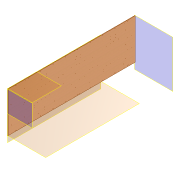
# Autodesk Inventor part: Top_Backboard
Saved by Autodesk Inventor 2018.1 (Build 221171000, 171)
## iProperties
Created: 2019-03-15
Part Number: Top_Backboard
Material: Wood (Cherry)
Document SubType Name: Modeling
Designer: James
Density: 0.63 g/cm^3
Appearance: Cherry - Natural Low Gloss
Mass: 60746.4 g
Surface Area: 108363 cm^2
Volume: 79929.5 cm^3
Author: James
Autodesk Inventor part; units mm, degrees
ref_plane "YZ Plane" through (0, 0, 0) normal (1, 0, 0) x (0, 1, 0)
ref_plane "XZ Plane" through (0, 0, 0) normal (0, 1, 0) x (-1, 0, 0)
ref_plane "XY Plane" through (0, 0, 0) normal (0, 0, 1) x (1, 0, 0)
derived "Top_Skeleton.ipt"
ref_plane "Work Plane1" through (0, 0, 0) normal (0, 0, 1) x (1, 0, 0)
ref_plane "Work Plane2" through (0, 0, 0) normal (0, 1, 0) x (-1, 0, 0)
ref_plane "Work Plane3" through (0, 0, 0) normal (1, 0, 0) x (0, 1, 0)
ref_plane "Work Plane4" through (0, 4100, 0) normal (0, 1, 0) x (-1, 0, 0)
ref_plane "Work Plane5" through (0, 0, -1300) normal (0, 0, 1) x (1, 0, 0)
sketch "Sketch2" plane through (0, 0, 0) normal (1, 0, 0) x (0, 1, 0)
  line L0 (0, 300) -> (0, -1800) projected
  line L1 (-820, 0) -> (4920, 0) projected
  line L2 (-820, -1300) -> (4920, -1300) projected
  line L3 (4100, 300) -> (4100, -1800) projected
  line L4 (0, 0) -> (4100, 0)
  line L5 (4100, 0) -> (4100, -1300)
  line L6 (4100, -1300) -> (0, -1300)
  line L7 (0, -1300) -> (0, 0)
  constraints: 8 end point, 4 point on line, 2 parallel, 1 horizontal, 1 perpendicular
extrude "Extrusion2" add sketch "Sketch2" along normal blind 15
sketch "Sketch3" plane through (15, 0, 0) normal (1, 0, 0) x (0, 0, -1)
  line L0 (1300, 4100) -> (0, 4100) projected
  line L1 (0, 4100) -> (0, 0) projected
  point P0 (487.5, 3991.5)
  point P1 (487.5, 3841.5)
  point P2 (822.5, 3841.5)
  point P3 (822.5, 3991.5)
  point P4 (487.5, 2881.3)
  point P5 (772.5, 2881.3)
  point P6 (772.5, 2731.3)
  point P7 (487.5, 2731.3)
  point P8 (487.5, 1771.1)
  point P9 (722.5, 1771.1)
  point P10 (722.5, 1621.1)
  point P11 (487.5, 1621.1)
  point P12 (487.5, 660.9)
  point P13 (672.5, 660.9)
  point P14 (672.5, 510.9)
  point P15 (487.5, 510.9)
  dimension "d7" = 150
  dimension "d8" = 335
  dimension "d16" = 150
  dimension "d17" = 150
  dimension "d18" = 150
  dimension "d19" = 285
  dimension "d20" = 235
  dimension "d21" = 185
  dimension "d22" = 108.5
  dimension "d23" = 487.5
  dimension "d24" = 1110.2
  dimension "d25" = 1110.2
  dimension "d26" = 1110.2
  constraints: 11 vertical alignment, 8 horizontal alignment
  measures "d7" distance of point (487.5, 3841.5) point (487.5, 3991.5)
  measures "d8" distance of point (822.5, 3991.5) point (487.5, 3991.5)
  measures "d16" distance of point (487.5, 2731.3) point (487.5, 2881.3)
  measures "d17" distance of point (487.5, 1621.1) point (487.5, 1771.1)
  measures "d18" distance of point (487.5, 510.9) point (487.5, 660.9)
  measures "d19" distance of point (772.5, 2881.3) point (487.5, 2881.3)
  measures "d20" distance of point (722.5, 1771.1) point (487.5, 1771.1)
  measures "d21" distance of point (672.5, 660.9) point (487.5, 660.9)
  measures "d22" distance from line of L0 point (487.5, 3991.5)
  measures "d23" distance from line of L1 point (487.5, 3991.5)
  measures "d24" vertical distance of point (772.5, 2881.3) point (822.5, 3991.5)
  measures "d25" vertical distance of point (722.5, 1771.1) point (772.5, 2881.3)
  measures "d26" vertical distance of point (672.5, 660.9) point (722.5, 1771.1)
hole "Selection Holes" at (15, 3991.5, -487.5) at (15, 3841.5, -487.5) at (15, 3841.5, -822.5) at (15, 3991.5, -822.5) at (15, 2881.3, -772.5) at (15, 2731.3, -772.5) at (15, 2731.3, -487.5) at (15, 2881.3, -487.5) at (15, 1771.1, -487.5) at (15, 1621.1, -487.5) at (15, 1621.1, -722.5) at (15, 1771.1, -722.5) at (15, 660.9, -487.5) at (15, 660.9, -672.5) at (15, 510.9, -672.5) at (15, 510.9, -487.5) direction (-1, 0, 0) diameter 4.5 end through all clearance for "Flat Head Machine Screw" size "M4" standard "Ansi Metric M Profile"
sketch "Sketch4" plane through (15, 0, 0) normal (1, 0, 0) x (0, 0, -1)
  circle A0 centre (672.5, 510.9) radius 2.25 projected
  circle A1 centre (487.5, 660.9) radius 2.25 projected
  circle A2 centre (722.5, 1621.1) radius 2.25 projected
  circle A3 centre (487.5, 1771.1) radius 2.25 projected
  circle A4 centre (487.5, 2731.3) radius 2.25 projected
  circle A5 centre (772.5, 2881.3) radius 2.25 projected
  circle A6 centre (822.5, 3841.5) radius 2.25 projected
  circle A7 centre (487.5, 3991.5) radius 2.25 projected
  circle A8 centre (487.5, 3841.5) radius 2.25 projected
  circle A9 centre (822.5, 3991.5) radius 2.25 projected
  circle A10 centre (772.5, 2731.3) radius 2.25 projected
  circle A11 centre (487.5, 2881.3) radius 2.25 projected
  circle A12 centre (487.5, 1621.1) radius 2.25 projected
  circle A13 centre (722.5, 1771.1) radius 2.25 projected
  circle A14 centre (672.5, 660.9) radius 2.25 projected
  circle A15 centre (487.5, 510.9) radius 2.25 projected
  line L0 (0, 0) -> (1300, 0) projected
  line L1 (1300, 0) -> (1300, 4100) projected
  line L2 (1300, 4100) -> (0, 4100) projected
  line L3 (0, 4100) -> (0, 0) projected
  point P0 (380, 3563)
  point P1 (935, 3563)
  point P2 (935, 3413)
  point P3 (380, 3413)
  point P4 (425, 2452.5)
  point P5 (885, 2452.5)
  point P6 (885, 2302.5)
  point P7 (425, 2302.5)
  point P8 (470, 1342.5)
  point P9 (835, 1342.5)
  point P10 (835, 1192.5)
  point P11 (470, 1192.5)
  dimension "d27" = 150
  dimension "d28" = 150
  dimension "d29" = 150
  dimension "d30" = 380
  dimension "d31" = 425
  dimension "d32" = 470
  dimension "d33" = 460
  dimension "d34" = 365
  dimension "d35" = 555
  dimension "d43" = 537
  dimension "d49" = 1110.5
  dimension "d50" = 1110
  constraints: 6 horizontal alignment, 6 vertical alignment
  measures "d27" distance of point (835, 1192.5) point (835, 1342.5)
  measures "d28" distance of point (885, 2452.5) point (885, 2302.5)
  measures "d29" distance of point (935, 3563) point (935, 3413)
  measures "d30" distance from line of L3 point (380, 3563)
  measures "d31" distance from line of point (425, 2452.5) L3
  measures "d32" distance from line of point (470, 1342.5) L3
  measures "d33" distance of point (885, 2452.5) point (425, 2452.5)
  measures "d34" distance of point (835, 1342.5) point (470, 1342.5)
  measures "d35" distance of point (935, 3563) point (380, 3563)
  measures "d43" distance from line of L2 point (935, 3563)
  measures "d49" vertical distance of point (885, 2452.5) point (935, 3563)
  measures "d50" vertical distance of point (835, 1342.5) point (885, 2452.5)
hole "Pancake Holes" at (15, 3563, -380) at (15, 3563, -935) at (15, 3413, -935) at (15, 3413, -380) at (15, 2452.5, -425) at (15, 2452.5, -885) at (15, 2302.5, -885) at (15, 2302.5, -425) at (15, 1342.5, -470) at (15, 1342.5, -835) at (15, 1192.5, -835) at (15, 1192.5, -470) direction (-1, 0, 0) diameter 4.5 end through all clearance for "Flat Head Machine Screw" size "M4" standard "Ansi Metric M Profile"
pattern_linear "Rectangular Pattern1" count 2 spacing 250 along (0, -1, 0) of "Pancake Holes"
sketch "Sketch5" plane through (15, 0, 0) normal (1, 0, 0) x (0, 0, -1)
  line L0 (1300, 0) -> (1300, 4100) projected
  line L1 (0, 4100) -> (0, 0) projected
  line L2 (-260, 4100) -> (1560, 4100) projected
  point P0 (25, 3850)
  point P1 (1275, 3850)
  dimension "d51" = 25
  dimension "d52" = 25
  dimension "d53" = 250
  constraints: 1 horizontal alignment
  measures "d51" distance from line of L0 point (1275, 3850)
  measures "d52" distance from line of L1 point (25, 3850)
  measures "d53" distance from line of point (25, 3850) L2
hole "Hole3" at (15, 3850, -25) at (15, 3850, -1275) direction (-1, 0, 0) diameter 4.496 end through all countersink diameter 8.433 countersink angle 82 clearance for "Flat Head Machine Screw (82)" size "#8" standard "Ansi Unified Screw Threads"
pattern_linear "Rectangular Pattern2" count 10 spacing 400 along (0, -1, 0) of "Hole3"
sketch "Sketch6" plane through (15, 0, 0) normal (1, 0, 0) x (0, 0, -1)
  line L0 (0, 4100) -> (0, 0) projected
  line L1 (-260, 4100) -> (1560, 4100) projected
  point P0 (250, 3800)
  point P1 (250, 2170)
  point P2 (250, 540)
  dimension "d64" = 250
  dimension "d65" = 300
  dimension "d76" = 1630
  dimension "d77" = 1630
  constraints: 2 vertical alignment
  measures "d64" distance from line of point (250, 3800) L0
  measures "d65" distance from line of point (250, 3800) L1
  measures "d76" distance of point (250, 2170) point (250, 3800)
  measures "d77" distance of point (250, 540) point (250, 2170)
hole "Hole4" at (15, 3800, -250) at (15, 2170, -250) at (15, 540, -250) direction (-1, 0, 0) diameter 4.496 end through all countersink diameter 8.433 countersink angle 82 clearance for "Flat Head Machine Screw (82)" size "#8" standard "Ansi Unified Screw Threads"
pattern_linear "Rectangular Pattern3" count 3 spacing 400 along (0, 0, -1) of "Hole4"
sketch "Sketch7" plane through (15, 0, 0) normal (1, 0, 0) x (0, 0, -1)
  circle A0 centre (1050, 2170) radius 4.2165 projected
  circle A1 centre (1050, 540) radius 4.2165 projected
  circle A2 centre (1050, 3800) radius 4.2165 projected
  circle A3 centre (650, 2170) radius 4.2165 projected
  circle A4 centre (650, 540) radius 4.2165 projected
  circle A5 centre (650, 3800) radius 4.2165 projected
  circle A6 centre (250, 2170) radius 4.2165 projected
  circle A7 centre (250, 3800) radius 4.2165 projected
  circle A8 centre (250, 540) radius 4.2165 projected
  circle A9 centre (25, 250) radius 4.2165 projected
  circle A10 centre (1275, 250) radius 4.2165 projected
  circle A11 centre (25, 650) radius 4.2165 projected
  circle A12 centre (1275, 650) radius 4.2165 projected
  circle A13 centre (25, 1050) radius 4.2165 projected
  circle A14 centre (1275, 1050) radius 4.2165 projected
  circle A15 centre (25, 1450) radius 4.2165 projected
  circle A16 centre (1275, 1450) radius 4.2165 projected
  circle A17 centre (25, 1850) radius 4.2165 projected
  circle A18 centre (1275, 1850) radius 4.2165 projected
  circle A19 centre (25, 2250) radius 4.2165 projected
  circle A20 centre (1275, 2250) radius 4.2165 projected
  circle A21 centre (25, 2650) radius 4.2165 projected
  circle A22 centre (1275, 2650) radius 4.2165 projected
  circle A23 centre (25, 3050) radius 4.2165 projected
  circle A24 centre (1275, 3050) radius 4.2165 projected
  circle A25 centre (25, 3450) radius 4.2165 projected
  circle A26 centre (1275, 3450) radius 4.2165 projected
  circle A27 centre (25, 3850) radius 4.2165 projected
  circle A28 centre (1275, 3850) radius 4.2165 projected
  circle A29 centre (835, 942.5) radius 2.25 projected
  circle A30 centre (470, 942.5) radius 2.25 projected
  circle A31 centre (835, 1092.5) radius 2.25 projected
  circle A32 centre (425, 2052.5) radius 2.25 projected
  circle A33 centre (885, 2202.5) radius 2.25 projected
  circle A34 centre (380, 3163) radius 2.25 projected
  circle A35 centre (935, 3313) radius 2.25 projected
  circle A36 centre (380, 3313) radius 2.25 projected
  circle A37 centre (935, 3163) radius 2.25 projected
  circle A38 centre (425, 2202.5) radius 2.25 projected
  circle A39 centre (885, 2052.5) radius 2.25 projected
  circle A40 centre (470, 1092.5) radius 2.25 projected
  circle A41 centre (835, 1192.5) radius 2.25 projected
  circle A42 centre (470, 1342.5) radius 2.25 projected
  circle A43 centre (885, 2302.5) radius 2.25 projected
  circle A44 centre (425, 2452.5) radius 2.25 projected
  circle A45 centre (935, 3413) radius 2.25 projected
  circle A46 centre (380, 3563) radius 2.25 projected
  circle A47 centre (935, 3563) radius 2.25 projected
  circle A48 centre (380, 3413) radius 2.25 projected
  circle A49 centre (885, 2452.5) radius 2.25 projected
  circle A50 centre (425, 2302.5) radius 2.25 projected
  circle A51 centre (835, 1342.5) radius 2.25 projected
  circle A52 centre (470, 1192.5) radius 2.25 projected
  circle A53 centre (672.5, 510.9) radius 2.25 projected
  circle A54 centre (487.5, 660.9) radius 2.25 projected
  circle A55 centre (722.5, 1621.1) radius 2.25 projected
  circle A56 centre (487.5, 1771.1) radius 2.25 projected
  circle A57 centre (487.5, 2731.3) radius 2.25 projected
  circle A58 centre (772.5, 2881.3) radius 2.25 projected
  circle A59 centre (822.5, 3841.5) radius 2.25 projected
  circle A60 centre (487.5, 3991.5) radius 2.25 projected
  circle A61 centre (487.5, 3841.5) radius 2.25 projected
  circle A62 centre (822.5, 3991.5) radius 2.25 projected
  circle A63 centre (772.5, 2731.3) radius 2.25 projected
  circle A64 centre (487.5, 2881.3) radius 2.25 projected
  circle A65 centre (487.5, 1621.1) radius 2.25 projected
  circle A66 centre (722.5, 1771.1) radius 2.25 projected
  circle A67 centre (672.5, 660.9) radius 2.25 projected
  circle A68 centre (487.5, 510.9) radius 2.25 projected
  line L0 (0, 0) -> (1300, 0) projected
  line L1 (1300, 0) -> (1300, 4100) projected
  line L2 (1300, 4100) -> (0, 4100) projected
  line L3 (0, 4100) -> (0, 0) projected
  point P0 (277.5, 3461.5)
  point P1 (277.5, 3311.5)
  point P2 (196.5, 3461.5)
  point P3 (196.5, 3311.5)
  point P4 (196.5, 2351.3)
  point P5 (277.5, 2351.3)
  point P6 (277.5, 2201.3)
  point P7 (196.5, 2201.3)
  point P8 (196.5, 1241.1)
  point P9 (277.5, 1241.1)
  point P10 (277.5, 1091.1)
  point P11 (196.5, 1091.1)
  dimension "d81" = 81
  dimension "d82" = 150
  dimension "d83" = 150
  dimension "d84" = 81
  dimension "d85" = 81
  dimension "d86" = 150
  dimension "d96" = 380
  dimension "d97" = 210
  dimension "d98" = 380
  dimension "d99" = 210
  dimension "d100" = 380
  dimension "d101" = 210
  constraints: 6 horizontal alignment, 6 vertical alignment
  measures "d81" distance of point (277.5, 3461.5) point (196.5, 3461.5)
  measures "d82" distance of point (196.5, 3311.5) point (196.5, 3461.5)
  measures "d83" distance of point (196.5, 2201.3) point (196.5, 2351.3)
  measures "d84" distance of point (277.5, 2351.3) point (196.5, 2351.3)
  measures "d85" distance of point (277.5, 1241.1) point (196.5, 1241.1)
  measures "d86" distance of point (196.5, 1241.1) point (196.5, 1091.1)
  measures "d96" vertical distance of point (277.5, 3461.5) A61.centre
  measures "d97" horizontal distance of A61.centre point (277.5, 3461.5)
  measures "d98" vertical distance of A57.centre point (277.5, 2351.3)
  measures "d99" horizontal distance of A57.centre point (277.5, 2351.3)
  measures "d100" vertical distance of A65.centre point (277.5, 1241.1)
  measures "d101" horizontal distance of A65.centre point (277.5, 1241.1)
hole "Hole5" at (15, 3461.5, -277.5) at (15, 3311.5, -277.5) at (15, 3461.5, -196.5) at (15, 3311.5, -196.5) at (15, 2351.3, -196.5) at (15, 2351.3, -277.5) at (15, 2201.3, -277.5) at (15, 2201.3, -196.5) at (15, 1241.1, -196.5) at (15, 1241.1, -277.5) at (15, 1091.1, -277.5) at (15, 1091.1, -196.5) direction (-1, 0, 0) diameter 4.5 end through all clearance for "Flat Head Machine Screw" size "M4" standard "Ansi Metric M Profile"
sketch "Sketch8" plane through (15, 0, 0) normal (1, 0, 0) x (0, 0, -1)
  circle A0 centre (277.5, 1091.1) radius 2.25 projected
  circle A1 centre (196.5, 1241.1) radius 2.25 projected
  circle A2 centre (277.5, 2201.3) radius 2.25 projected
  circle A3 centre (196.5, 2351.3) radius 2.25 projected
  circle A4 centre (196.5, 3461.5) radius 2.25 projected
  circle A5 centre (277.5, 3461.5) radius 2.25 projected
  circle A6 centre (277.5, 3311.5) radius 2.25 projected
  circle A7 centre (196.5, 3311.5) radius 2.25 projected
  circle A8 centre (277.5, 2351.3) radius 2.25 projected
  circle A9 centre (196.5, 2201.3) radius 2.25 projected
  circle A10 centre (277.5, 1241.1) radius 2.25 projected
  circle A11 centre (196.5, 1091.1) radius 2.25 projected
  circle A12 centre (1050, 2170) radius 4.2165 projected
  circle A13 centre (1050, 540) radius 4.2165 projected
  circle A14 centre (1050, 3800) radius 4.2165 projected
  circle A15 centre (650, 2170) radius 4.2165 projected
  circle A16 centre (650, 540) radius 4.2165 projected
  circle A17 centre (650, 3800) radius 4.2165 projected
  circle A18 centre (250, 2170) radius 4.2165 projected
  circle A19 centre (250, 3800) radius 4.2165 projected
  circle A20 centre (250, 540) radius 4.2165 projected
  circle A21 centre (25, 250) radius 4.2165 projected
  circle A22 centre (1275, 250) radius 4.2165 projected
  circle A23 centre (25, 650) radius 4.2165 projected
  circle A24 centre (1275, 650) radius 4.2165 projected
  circle A25 centre (25, 1050) radius 4.2165 projected
  circle A26 centre (1275, 1050) radius 4.2165 projected
  circle A27 centre (25, 1450) radius 4.2165 projected
  circle A28 centre (1275, 1450) radius 4.2165 projected
  circle A29 centre (25, 1850) radius 4.2165 projected
  circle A30 centre (1275, 1850) radius 4.2165 projected
  circle A31 centre (25, 2250) radius 4.2165 projected
  circle A32 centre (1275, 2250) radius 4.2165 projected
  circle A33 centre (25, 2650) radius 4.2165 projected
  circle A34 centre (1275, 2650) radius 4.2165 projected
  circle A35 centre (25, 3050) radius 4.2165 projected
  circle A36 centre (1275, 3050) radius 4.2165 projected
  circle A37 centre (25, 3450) radius 4.2165 projected
  circle A38 centre (1275, 3450) radius 4.2165 projected
  circle A39 centre (25, 3850) radius 4.2165 projected
  circle A40 centre (1275, 3850) radius 4.2165 projected
  circle A41 centre (835, 942.5) radius 2.25 projected
  circle A42 centre (470, 942.5) radius 2.25 projected
  circle A43 centre (835, 1092.5) radius 2.25 projected
  circle A44 centre (425, 2052.5) radius 2.25 projected
  circle A45 centre (885, 2202.5) radius 2.25 projected
  circle A46 centre (380, 3163) radius 2.25 projected
  circle A47 centre (935, 3313) radius 2.25 projected
  circle A48 centre (380, 3313) radius 2.25 projected
  circle A49 centre (935, 3163) radius 2.25 projected
  circle A50 centre (425, 2202.5) radius 2.25 projected
  circle A51 centre (885, 2052.5) radius 2.25 projected
  circle A52 centre (470, 1092.5) radius 2.25 projected
  circle A53 centre (835, 1192.5) radius 2.25 projected
  circle A54 centre (470, 1342.5) radius 2.25 projected
  circle A55 centre (885, 2302.5) radius 2.25 projected
  circle A56 centre (425, 2452.5) radius 2.25 projected
  circle A57 centre (935, 3413) radius 2.25 projected
  circle A58 centre (380, 3563) radius 2.25 projected
  circle A59 centre (935, 3563) radius 2.25 projected
  circle A60 centre (380, 3413) radius 2.25 projected
  circle A61 centre (885, 2452.5) radius 2.25 projected
  circle A62 centre (425, 2302.5) radius 2.25 projected
  circle A63 centre (835, 1342.5) radius 2.25 projected
  circle A64 centre (470, 1192.5) radius 2.25 projected
  circle A65 centre (672.5, 510.9) radius 2.25 projected
  circle A66 centre (487.5, 660.9) radius 2.25 projected
  circle A67 centre (722.5, 1621.1) radius 2.25 projected
  circle A68 centre (487.5, 1771.1) radius 2.25 projected
  circle A69 centre (487.5, 2731.3) radius 2.25 projected
  circle A70 centre (772.5, 2881.3) radius 2.25 projected
  circle A71 centre (822.5, 3841.5) radius 2.25 projected
  circle A72 centre (487.5, 3991.5) radius 2.25 projected
  circle A73 centre (487.5, 3841.5) radius 2.25 projected
  circle A74 centre (822.5, 3991.5) radius 2.25 projected
  circle A75 centre (772.5, 2731.3) radius 2.25 projected
  circle A76 centre (487.5, 2881.3) radius 2.25 projected
  circle A77 centre (487.5, 1621.1) radius 2.25 projected
  circle A78 centre (722.5, 1771.1) radius 2.25 projected
  circle A79 centre (672.5, 660.9) radius 2.25 projected
  circle A80 centre (487.5, 510.9) radius 2.25 projected
  line L0 (0, 0) -> (1300, 0) projected
  line L1 (1300, 0) -> (1300, 4100) projected
  line L2 (1300, 4100) -> (0, 4100) projected
  line L3 (0, 4100) -> (0, 0) projected
  point P0 (997, 3085.5)
  point P1 (1043, 3085.5)
  point P2 (947, 1974.5)
  point P3 (993, 1974.5)
  point P4 (897, 864.5)
  point P5 (943, 864.5)
  point P6 (747, 237)
  point P7 (793, 237)
  point P8 (872, 237)
  point P9 (918, 237)
  point P10 (997, 237)
  point P11 (1043, 237)
  point P12 (497, 237)
  point P13 (543, 237)
  point P14 (622, 237)
  point P15 (668, 237)
  dimension "d102" = 257
  dimension "d103" = 1014.5
  dimension "d104" = 46
  dimension "d105" = 46
  dimension "d106" = 46
  dimension "d107" = 46
  dimension "d108" = 46
  dimension "d109" = 46
  dimension "d110" = 2125.5
  dimension "d111" = 307
  dimension "d112" = 357
  dimension "d113" = 3235.5
  dimension "d121" = 3863
  dimension "d122" = 257
  dimension "d123" = 125
  dimension "d124" = 125
  dimension "d125" = 46
  dimension "d126" = 46
  dimension "d127" = 125
  dimension "d128" = 125
  constraints: 12 horizontal alignment
  measures "d102" distance from line of L1 point (1043, 3085.5)
  measures "d103" distance from line of L2 point (1043, 3085.5)
  measures "d104" distance of point (1043, 3085.5) point (997, 3085.5)
  measures "d105" distance of point (993, 1974.5) point (947, 1974.5)
  measures "d106" distance of point (943, 864.5) point (897, 864.5)
  measures "d107" distance of point (793, 237) point (747, 237)
  measures "d108" distance of point (918, 237) point (872, 237)
  measures "d109" distance of point (1043, 237) point (997, 237)
  measures "d110" distance from line of point (993, 1974.5) L2
  measures "d111" distance from line of point (993, 1974.5) L1
  measures "d112" distance from line of L1 point (943, 864.5)
  measures "d113" distance from line of L2 point (943, 864.5)
  measures "d121" distance from line of point (1043, 237) L2
  measures "d122" distance from line of point (1043, 237) L1
  measures "d123" distance of point (1043, 237) point (918, 237)
  measures "d124" distance of point (918, 237) point (793, 237)
  measures "d125" distance of point (668, 237) point (622, 237)
  measures "d126" distance of point (543, 237) point (497, 237)
  measures "d127" distance of point (747, 237) point (622, 237)
  measures "d128" distance of point (622, 237) point (497, 237)
hole "Hole6" at (15, 3085.5, -997) at (15, 3085.5, -1043) at (15, 1974.5, -947) at (15, 1974.5, -993) at (15, 864.5, -897) at (15, 864.5, -943) direction (-1, 0, 0) diameter 3.4 end through all clearance for "Flat Head Machine Screw" size "M3" standard "Ansi Metric M Profile"
sketch "Sketch9" plane through (15, 0, 0) normal (1, 0, 0) x (0, 0, -1)
  circle A0 centre (722.5, 1771.1) radius 2.25 projected
  point P0 (0, 0)
  point P1 (1172.5, 971.1)
  dimension "d129" = 450
  dimension "d130" = 800
  measures "d129" horizontal distance of A0.centre point (1172.5, 971.1)
  measures "d130" vertical distance of point (1172.5, 971.1) A0.centre
hole "Hole7" at (15, 971.1, -1172.5) direction (-1, 0, 0) diameter 9 end through all clearance for "Flat Head Machine Screw" size "M8" standard "Ansi Metric M Profile"
sketch "Sketch10" plane through (15, 0, 0) normal (1, 0, 0) x (0, 0, -1)
  circle A0 centre (1172.5, 971.1) radius 4.5 projected
  circle A1 centre (822.5, 3841.5) radius 2.25 projected
  circle A2 centre (772.5, 2731.3) radius 2.25 projected
  circle A3 centre (722.5, 1621.1) radius 2.25 projected
  point P0 (0, 0)
  point P1 (1072.5, 1171.1)
  point P2 (1112.5, 1171.1)
  point P3 (1152.5, 1171.1)
  point P4 (730, 1531.1)
  point P5 (780, 2641.3)
  point P6 (830, 3751.5)
  point P7 (1059.5, 1501.1)
  point P8 (1085.5, 1501.1)
  point P9 (1096.5, 2611.3)
  point P10 (1122.5, 2611.3)
  point P11 (1136.5, 3721.5)
  point P12 (1162.5, 3721.5)
  dimension "d138" = 100
  dimension "d139" = 40
  dimension "d140" = 40
  dimension "d141" = 200
  dimension "d149" = 90
  dimension "d150" = 7.5
  dimension "d151" = 90
  dimension "d152" = 7.5
  dimension "d153" = 90
  dimension "d154" = 7.5
  dimension "d155" = 26
  dimension "d156" = 26
  dimension "d157" = 26
  dimension "d158" = 13
  dimension "d159" = 16
  dimension "d160" = 10
  dimension "d161" = 30
  dimension "d162" = 30
  dimension "d163" = 30
  constraints: 5 horizontal alignment
  measures "d138" horizontal distance of A0.centre point (1072.5, 1171.1)
  measures "d139" distance of point (1072.5, 1171.1) point (1112.5, 1171.1)
  measures "d140" distance of point (1152.5, 1171.1) point (1112.5, 1171.1)
  measures "d141" vertical distance of A0.centre point (1152.5, 1171.1)
  measures "d149" vertical distance of point (730, 1531.1) A3.centre
  measures "d150" horizontal distance of A3.centre point (730, 1531.1)
  measures "d151" vertical distance of point (780, 2641.3) A2.centre
  measures "d152" horizontal distance of point (780, 2641.3) A2.centre
  measures "d153" vertical distance of A1.centre point (830, 3751.5)
  measures "d154" horizontal distance of point (830, 3751.5) A1.centre
  measures "d155" distance of point (1085.5, 1501.1) point (1059.5, 1501.1)
  measures "d156" distance of point (1122.5, 2611.3) point (1096.5, 2611.3)
  measures "d157" distance of point (1162.5, 3721.5) point (1136.5, 3721.5)
  measures "d158" horizontal distance of point (1059.5, 1501.1) point (1072.5, 1171.1)
  measures "d159" horizontal distance of point (1112.5, 1171.1) point (1096.5, 2611.3)
  measures "d160" horizontal distance of point (1152.5, 1171.1) point (1162.5, 3721.5)
  measures "d161" vertical distance of point (730, 1531.1) point (1059.5, 1501.1)
  measures "d162" vertical distance of point (780, 2641.3) point (1096.5, 2611.3)
  measures "d163" vertical distance of point (830, 3751.5) point (1136.5, 3721.5)
hole "Hole8" at (15, 1171.1, -1072.5) at (15, 1171.1, -1112.5) at (15, 1171.1, -1152.5) at (15, 1531.1, -730) at (15, 2641.3, -780) at (15, 3751.5, -830) at (15, 1501.1, -1059.5) at (15, 1501.1, -1085.5) at (15, 2611.3, -1096.5) at (15, 2611.3, -1122.5) at (15, 3721.5, -1136.5) at (15, 3721.5, -1162.5) direction (-1, 0, 0) diameter 3.4 end through all clearance for "Flat Head Machine Screw" size "M3" standard "Ansi Metric M Profile"
sketch "Sketch11" plane through (15, 0, 0) normal (1, 0, 0) x (0, 0, -1)
  line L0 (-260, 4100) -> (1560, 4100) projected
  line L1 (0, 4100) -> (0, 0) projected
  line L2 (1300, 0) -> (1300, 4100) projected
  point P0 (27.5, 3900)
  point P1 (27.5, 3750)
  point P2 (1272.5, 3900)
  point P3 (1272.5, 3750)
  dimension "d164" = 200
  dimension "d165" = 150
  dimension "d166" = 27.5
  dimension "d167" = 27.5
  constraints: 2 horizontal alignment, 2 vertical alignment
  measures "d164" distance from line of L0 point (27.5, 3900)
  measures "d165" distance of point (27.5, 3750) point (27.5, 3900)
  measures "d166" distance from line of point (27.5, 3900) L1
  measures "d167" distance from line of L2 point (1272.5, 3900)
hole "Hole9" at (15, 3900, -27.5) at (15, 3750, -27.5) at (15, 3900, -1272.5) at (15, 3750, -1272.5) direction (-1, 0, 0) diameter 3.302 depth 12.3 tip angle 118 thread size "8-32 UNC" class "2B" standard "ANSI Unified Screw Threads"
pattern_linear "Rectangular Pattern4" count 3 spacing 1600 along (0, -1, 0) of "Hole9"
sketch "Sketch12" plane through (15, 0, 0) normal (1, 0, 0) x (0, 0, -1)
  circle A0 centre (497, 237) radius 1.7 projected
  circle A1 centre (1043, 237) radius 1.7 projected
  line L0 (-260, 0) -> (1560, 0) projected
  circle A2 centre (487.5, 510.9) radius 2.25 projected
  point P0 (0, 0)
  point P1 (482.5, 117)
  point P2 (482.5, 92)
  point P3 (1057.5, 117)
  point P4 (1057.5, 92)
  dimension "d178" = 25
  dimension "d183" = 92
  dimension "d184" = 575
  dimension "d185" = 5
  constraints: 2 horizontal alignment, 2 vertical alignment
  measures "d178" distance of point (1057.5, 92) point (1057.5, 117)
  measures "d183" distance from line of point (482.5, 92) L0
  measures "d184" distance of point (1057.5, 117) point (482.5, 117)
  measures "d185" horizontal distance of A2.centre point (482.5, 117)
hole "Hole10" at (15, 117, -482.5) at (15, 92, -482.5) at (15, 117, -1057.5) at (15, 92, -1057.5) direction (-1, 0, 0) diameter 4.5 end through all clearance for "Flat Head Machine Screw" size "M4" standard "Ansi Metric M Profile"
equation "\"d16\" = d7"
equation "\"d17\" = d16"
equation "\"d18\" = d17"
equation "\"d25\" = d24"
equation "\"d26\" = d24"
equation "\"d28\" = d27"
equation "\"d29\" = d28"
equation "\"d52\" = d51"
equation "\"d77\" = d76"
equation "\"d83\" = d82"
equation "\"d84\" = d81"
equation "\"d85\" = d84"
equation "\"d86\" = d83"
equation "\"d98\" = d96"
equation "\"d99\" = d97"
equation "\"d100\" = d98"
equation "\"d101\" = d99"
equation "\"d105\" = d104"
equation "\"d106\" = d105"
equation "\"d107\" = d106"
equation "\"d108\" = d107"
equation "\"d109\" = d108"
equation "\"d124\" = d123"
equation "\"d125\" = d107"
equation "\"d126\" = d125"
equation "\"d127\" = d124"
equation "\"d128\" = d127"
equation "\"d140\" = d139"
equation "\"d153\" = d151"
equation "\"d154\" = d152"
equation "\"d156\" = d155"
equation "\"d157\" = d155"
equation "\"d158\" = 0.5 * d155"
equation "\"d167\" = d166"
body "Solid2"
